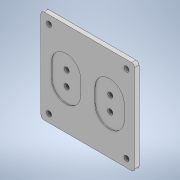
# Autodesk Inventor part: ジンバル1-1
Saved by Autodesk Inventor 2020 (Build 240168000, 168)
## iProperties
Created: 2019-11-07
Part Number: ジンバル1-1
Material: 一般
Document SubType Name: Modeling
Designer: highs
Density: 1 g/cm^3
Appearance: 既定
Author: highs
## iProperties of the stored document _3D プリント.ipt
Created: 2019-11-07
Part Number: _3D プリント
Material: 一般
Document SubType Name: Modeling
Designer: highs
Density: 1 g/cm^3
Appearance: 既定
Author: highs
Autodesk Inventor part; units mm, degrees
ref_plane "YZ Plane" through (0, 0, 0) normal (1, 0, 0) x (0, 1, 0)
ref_plane "XZ Plane" through (0, 0, 0) normal (0, 1, 0) x (-1, 0, 0)
ref_plane "XY Plane" through (0, 0, 0) normal (0, 0, 1) x (1, 0, 0)
sketch "スケッチ1" plane through (0, 0, 0) normal (0, 0, 1) x (1, 0, 0)
  line L0 (0, 0) -> (64, 0)
  line L1 (64, 0) -> (64, 64)
  line L2 (64, 64) -> (0, 64)
  line L3 (0, 64) -> (0, 0)
  line L4 (5.5, 58.5) -> (58.5, 58.5) construction
  line L5 (58.5, 58.5) -> (58.5, 5.5) construction
  line L6 (58.5, 5.5) -> (5.5, 5.5) construction
  line L7 (5.5, 5.5) -> (5.5, 58.5) construction
  circle A0 centre (5.5, 58.5) radius 1.75
  circle A1 centre (5.5, 5.5) radius 1.75
  circle A2 centre (58.5, 5.5) radius 1.75
  circle A3 centre (58.5, 58.5) radius 1.75
  line L8 (0, 32) -> (64, 32) construction
  line L9 (32, 64) -> (32, 0) construction
  line L10 (17.1, 27.05) -> (46.9, 27.05) construction
  line L11 (46.9, 27.05) -> (46.9, 36.95) construction
  line L12 (46.9, 36.95) -> (17.1, 36.95) construction
  line L13 (17.1, 36.95) -> (17.1, 27.05) construction
  line L14 (17.1, 27.05) -> (46.9, 36.95) construction
  line L15 (46.9, 27.05) -> (17.1, 36.95) construction
  circle A4 centre (46.9, 36.95) radius 1.75
  circle A5 centre (46.9, 27.05) radius 1.75
  circle A6 centre (17.1, 27.05) radius 1.75
  circle A7 centre (17.1, 36.95) radius 1.75
  point P0 (32, 32)
  dimension "d0" = 64
  dimension "d2" = 53
  dimension "d3" = 3.5
  dimension "d4" = 3.5
  dimension "d5" = 9.9
  dimension "d6" = 29.8
  constraints: 32 end point, 8 centre point, 8 coincident, 7 midpoint, 6 equal radius, 6 parallel, 4 perpendicular, 2 horizontal, 3 other
  measures "d0" distance of L0.start L0.end
  measures "d2" distance of L5.end L6.end
  measures "d3" diameter of A3
  measures "d4" diameter of A7
  measures "d5" distance of L12.end L10.start
  measures "d6" distance of L11.end L12.end
extrude "押し出し1" add sketch "スケッチ1" along normal blind 3
fillet "フィレット1" radius 2 4 edges at (0, 0, 1.5) (64, 0, 1.5) (64, 64, 1.5) (0, 64, 1.5)
sketch "スケッチ2" plane through (0, 0, 3) normal (0, 0, 1) x (1, 0, 0)
  circle A0 centre (17.1, 36.95) radius 1.75 projected
  circle A1 centre (17.1, 27.05) radius 1.75 projected
  line L0 (17.1, 36.95) -> (17.1, 27.05) construction
  line L1 (7.1, 36.95) -> (7.1, 27.05)
  line L2 (27.1, 27.05) -> (27.1, 36.95)
  arc A2 (27.1, 36.95) -> (7.1, 36.95) centre (17.1, 36.95) ccw
  arc A3 (7.1, 27.05) -> (27.1, 27.05) centre (17.1, 27.05) ccw
  circle A4 centre (46.9, 36.95) radius 1.75 projected
  circle A5 centre (46.9, 27.05) radius 1.75 projected
  line L3 (46.9, 36.95) -> (46.9, 27.05) construction
  line L4 (36.9, 36.95) -> (36.9, 27.05)
  line L5 (56.9, 27.05) -> (56.9, 36.95)
  arc A6 (56.9, 36.95) -> (36.9, 36.95) centre (46.9, 36.95) ccw
  arc A7 (36.9, 27.05) -> (56.9, 27.05) centre (46.9, 27.05) ccw
  point P0 (0, 0)
  point P1 (17.1, 32)
  point P2 (46.9, 32)
  dimension "d10" = 10
  dimension "d11" = 10
  constraints: 16 end point, 8 point on circle, 8 tangent, 4 centre point, 3 parallel, 2 midpoint, 1 vertical
  measures "d10" radius of A2
  measures "d11" radius of A6
extrude "押し出し2" cut sketch "スケッチ2" against normal blind 0.5
